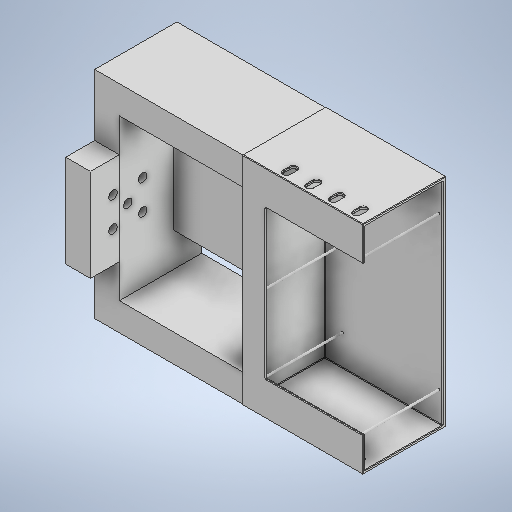
# Autodesk Inventor part: Intake_I2D_Bottom
Saved by Autodesk Inventor 2025 (Build 290162010, 162A)
## iProperties
Created: 2024-10-13
Part Number: Intake_I2D_Bottom
Material: Generic
Document SubType Name: Modeling
Designer: dcfam
Density: 1 g/cm^3
Appearance: Default
Author: dcfam
Autodesk Inventor part; units mm, degrees
ref_plane "YZ Plane" through (0, 0, 0) normal (1, 0, 0) x (0, 1, 0)
ref_plane "XZ Plane" through (0, 0, 0) normal (0, 1, 0) x (-1, 0, 0)
ref_plane "XY Plane" through (0, 0, 0) normal (0, 0, 1) x (1, 0, 0)
sketch "Sketch1" plane through (0, 0, 0) normal (0, 0, 1) x (1, 0, 0)
  line L0 (-32.5, -58.5) -> (32.5, -58.5)
  line L1 (32.5, -58.5) -> (32.5, 58.5)
  line L2 (32.5, 58.5) -> (-32.5, 58.5)
  line L3 (-32.5, 58.5) -> (-32.5, -58.5)
  line L4 (-32.5, -58.5) -> (32.5, 58.5) construction
  line L5 (32.5, -58.5) -> (-32.5, 58.5) construction
  point P0 (0, 0)
  dimension "d0" = 65
  dimension "d1" = 117
  constraints: 12 end point, 2 midpoint, 2 parallel, 1 horizontal, 1 perpendicular
  measures "d0" distance of L2.end L1.end
  measures "d1" distance of L1.end L0.end
extrude "Extrusion1" add sketch "Sketch1" along normal blind 2
sketch "Sketch2" plane through (0, 0, 2) normal (0, 0, 1) x (1, 0, 0)
  line L0 (32.5, -58.5) -> (32.5, 58.5) projected
  line L1 (32.5, 58.5) -> (-32.5, 58.5) projected
  line L2 (-32.5, 58.5) -> (-32.5, -58.5) projected
  line L3 (-32.5, -58.5) -> (32.5, -58.5) projected
  line L4 (31, 57) -> (-31, 57)
  line L5 (-31, 57) -> (-31, -57)
  line L6 (-31, -57) -> (26, -57)
  line L7 (26, -57) -> (32.5, -57)
  line L8 (32.5, -58.5) -> (32.5, 58.5) projected
  line L9 (32.5, -57) -> (32.5, -58.5)
  line L10 (31, 57) -> (32.5, 57)
  line L11 (32.5, 57) -> (32.5, 58.5)
  line L12 (32.5, 58.5) -> (-32.5, 58.5)
  line L13 (-32.5, 58.5) -> (-32.5, -58.5)
  line L14 (-32.5, -58.5) -> (32.5, -58.5)
  point P0 (0, 0)
  dimension "d4" = 1.5
  constraints: 20 end point, 4 perpendicular, 2 collinear, 2 point on line, 1 horizontal, 2 other
  measures "d4" distance between parallel lines of L3 L6
extrude "Extrusion2" add sketch "Sketch2" along normal blind 43 contours L3 L2 L1 L0 L10 L4 L5 L6 L7
sketch "Sketch3" plane through (0, 0, 45) normal (0, 0, 1) x (1, 0, 0)
  line L0 (-32.5, -58.5) -> (32.5, -58.5) projected
  line L1 (32.5, 58.5) -> (-32.5, 58.5) projected
  line L2 (-32.5, -58.5) -> (32.5, -58.5)
  line L3 (32.5, -58.5) -> (32.5, 58.5)
  line L4 (32.5, 58.5) -> (-32.5, 58.5)
  line L5 (-32.5, 58.5) -> (-32.5, -58.5)
  point P0 (0, 0)
  constraints: 8 end point, 2 parallel, 1 horizontal, 1 perpendicular
extrude "Extrusion3" add sketch "Sketch3" against normal blind 1
sketch "Sketch4" plane through (0, 0, 45) normal (0, 0, 1) x (1, 0, 0)
  line L0 (20, -40) -> (-20, -40)
  line L1 (-20, -40) -> (-20, 40)
  line L2 (-20, 40) -> (20, 40)
  line L3 (20, -40) -> (-20, 40) construction
  line L4 (-20, -40) -> (20, 40) construction
  line L5 (20, -40) -> (32.5, -40)
  line L6 (32.5, 57) -> (32.5, -57) projected
  line L7 (20, 40) -> (32.5, 40)
  line L8 (32.5, 40) -> (32.5, -40)
  line L9 (32.5, -40) -> (32.5, 40)
  point P0 (0, 0)
  point P1 (32.5, 40)
  dimension "d9" = 40
  dimension "d10" = 80
  constraints: 18 end point, 3 horizontal, 2 midpoint, 2 perpendicular, 1 collinear, 1 parallel, 1 point on line
  measures "d9" distance of L1.end L2.end
  measures "d10" distance of L0.end L1.end
extrude "Extrusion4" cut sketch "Sketch4" against normal blind 10.525
sketch "Sketch5" plane through (-32.5, 58.5, 0) normal (0, 1, 0) x (1, 0, 0)
  arc A0 (59.7, -37.9468) -> (56.3, -37.9468) centre (58, -37.7472) ccw
  line L0 (56.3, -37.9468) -> (56.3, -41.0568)
  line L1 (56.3, -41.0568) -> (56.3, -37.9468)
  line L2 (56.3, -39.5018) -> (63.0274, -39.5018) construction
  arc A1 (56.3, -41.0568) -> (59.7, -41.0568) centre (58, -41.2563) ccw
  line L3 (58, -41.2563) -> (58, -37.7472) construction
  line L4 (59.7, -37.9468) -> (59.7, -41.0568)
  line L5 (65, 0) -> (65, -45) construction
  line L6 (65, 0) -> (0, 0) construction
  line L7 (0, 0) -> (0, -45) construction
  line L8 (65, -45) -> (0, -45) construction
  arc A2 (43.7, -41.0568) -> (47.1, -41.0568) centre (45.4, -41.2563) ccw
  line L9 (47.1, -37.9468) -> (47.1, -41.0568)
  arc A3 (47.1, -37.9468) -> (43.7, -37.9468) centre (45.4, -37.7472) ccw
  line L10 (43.7, -37.9468) -> (43.7, -41.0568)
  arc A4 (31.1, -41.0568) -> (34.5, -41.0568) centre (32.8, -41.2563) ccw
  line L11 (34.5, -37.9468) -> (34.5, -41.0568)
  arc A5 (34.5, -37.9468) -> (31.1, -37.9468) centre (32.8, -37.7472) ccw
  line L12 (31.1, -37.9468) -> (31.1, -41.0568)
  arc A6 (18.5, -41.0568) -> (21.9, -41.0568) centre (20.2, -41.2563) ccw
  line L13 (21.9, -37.9468) -> (21.9, -41.0568)
  arc A7 (21.9, -37.9468) -> (18.5, -37.9468) centre (20.2, -37.7472) ccw
  line L14 (18.5, -37.9468) -> (18.5, -41.0568)
  line L15 (58, -42.968) -> (20.2, -42.968) construction
  line L16 (39.1, -42.968) -> (39.1, -55.668) construction
  point P0 (32.5, 0)
  point P1 (21.9, -37.9468)
  point P2 (18.5, -41.0568)
  point P3 (21.9, -41.0568)
  point P4 (34.5, -37.9468)
  point P5 (31.1, -41.0568)
  point P6 (34.5, -41.0568)
  point P7 (47.1, -37.9468)
  point P8 (43.7, -41.0568)
  point P9 (47.1, -41.0568)
  point P10 (59.7, -37.9468)
  point P11 (56.3, -41.0568)
  point P12 (59.7, -41.0568)
  dimension "d13" = 3.4
  dimension "d14" = 1.7117
  dimension "d15" = 3.11
  dimension "d16" = 3.11
  dimension "d19" = 12.6
  dimension "d24" = 2.032
  dimension "d37" = 12.7
  dimension "d47" = 32.6288
  dimension "d48" = 1.9726
  dimension "d49" = 1.9726
  dimension "d50" = 35.7388
  dimension "d51" = 1.9726
  dimension "d52" = 35.7388
  dimension "d53" = 5.3726
  dimension "d54" = 32.6288
  dimension "d55" = 14.5726
  dimension "d56" = 35.7388
  dimension "d57" = 14.5726
  dimension "d58" = 35.7388
  dimension "d59" = 17.9726
  dimension "d60" = 32.6288
  dimension "d61" = 27.1726
  dimension "d62" = 35.7388
  dimension "d63" = 27.1726
  dimension "d64" = 35.7388
  dimension "d65" = 30.5726
  dimension "d66" = 32.6288
  dimension "d67" = 39.7726
  dimension "d68" = 35.7388
  dimension "d69" = 39.7726
  dimension "d70" = 35.7388
  dimension "d71" = 43.1726
  dimension "d84" = 5.3
  constraints: 26 end point, 18 point on circle, 8 centre point, 5 symmetric about line, 4 point on line, 3 vertical, 2 horizontal, 2 midpoint, 1 coincident, 1 tangent, 43 other
  measures "d13" distance of A0.start L0.start
  measures "d14" radius of A0
  measures "d15" distance of L0.start L0.end
  measures "d16" distance of L0.end L1.end
  measures "d19" distance of L3.start A2.centre
  measures "d24" distance from line of L8 L15.start
  measures "d37" distance of L16.start L16.end
  measures "d49" distance from line of L2.end L5
  measures "d84" distance between parallel lines of L5 L4
extrude "Extrusion5" cut sketch "Sketch5" against normal blind 25.4
sketch "Sketch6" plane through (-32.5, -58.5, 0) normal (0, -1, 0) x (1, 0, 0)
  circle A0 centre (57.992, 40.3585) radius 1.9625
  line L0 (0, 0) -> (0, 45) projected
  line L1 (0, 0) -> (65, 0) projected
  line L2 (65, 0) -> (65, 45) projected
  line L3 (0, 45) -> (65, 45) projected
  circle A1 centre (49.991, 40.3585) radius 1.9625
  circle A2 centre (41.99, 40.3585) radius 1.9625
  circle A3 centre (33.989, 40.3585) radius 1.9625
  line L4 (33.989, 42.321) -> (57.992, 42.321) construction
  line L5 (45.9905, 42.321) -> (45.9905, 58.396) construction
  point P0 (32.5, 0)
  dimension "d27" = 3.925
  dimension "d30" = 8.001
  dimension "d35" = 2.679
  dimension "d36" = 16.075
  dimension "d87" = 7.008
  constraints: 4 end point, 2 centre point, 2 horizontal, 2 vertical alignment, 1 coincident, 1 midpoint, 1 vertical, 10 other
  measures "d30" distance of point (57.992, 40.358) A1.centre
  measures "d35" distance between parallel lines of L3 L4
  measures "d36" distance of L5.start L5.end
  measures "d87" distance from line of L2 point (57.992, 40.358)
extrude "Extrusion6" cut sketch "Sketch6" against normal blind 25.4 contours A0 | A1 | A2 | A3
chamfer "Chamfer1" distance 0.5 angle 45 8 edges at (23.5295, -57, 40.3585) (15.5285, -57, 40.3585) (7.5275, -57, 40.3585) (-0.4735, -57, 40.3585) (-0.4735, -58.5, 40.3585) (7.5275, -58.5, 40.3585) (15.5285, -58.5, 40.3585) (23.5295, -58.5, 40.3585)
fillet "Fillet1" radius 0.3 100 edges at (0, -58.5, 45) (15.5285, -57.5, 40.3585) (15.0285, -57, 40.3585) (23.5295, -58, 40.3585) (23.5295, -57.5, 40.3585) (23.0295, -58.5, 40.3585) (7.0275, -58.5, 40.3585) (23.0295, -57, 40.3585) (7.0275, -57, 40.3585) (-0.4735, -58, 40.3585) (-0.4735, -57.5, 40.3585) (-0.9735, -58.5, 40.3585) (-0.9735, -57, 40.3585) (32.5, -57, 23) (32.5, -58.5, 22.5) (0.75, -57, 44) (0.75, -57, 2) (0, -58.5, 0) (-31, -57, 23) (-32.5, -58.5, 22.5) (7.5275, -58, 40.3585) (15.5285, -58, 40.3585) (15.0285, -58.5, 40.3585) (7.5275, -57.5, 40.3585) (-20, 0, 44) (-20, 0, 45) (-31, 0, 44) (-32.5, 0, 45) (-32.5, 0, 0) (0.75, 57, 44) (0.75, 57, 2) (-31, 57, 23) (0, 58.5, 45) (0, 58.5, 0) (-32.5, 58.5, 22.5) (32.5, 57, 23) (32.5, 49.25, 45) (32.5, 58.5, 22.5) (32.5, 48.5, 44) (32.5, -48.5, 44) (32.5, 0, 0) (32.5, 0, 2) (32.5, -49.25, 45) (6.25, -40, 45) (6.25, -40, 44) (32.5, -40, 44.5) (-20, -40, 44.5) (-31, 0, 2) (32.5, 40, 44.5) (-20, 40, 44.5) (6.25, 40, 45) (6.25, 40, 44) (27.2, 58.5, 39.5018) (23.8, 57, 39.5018) (27.2, 57, 39.5018) (25.5, 57, 36.0355) (25.5, 57, 42.968) (23.8, 58.5, 39.5018) (23.8, 57.75, 37.9468) (25.5, 58.5, 36.0355) (27.2, 57.75, 37.9468) (27.2, 57.75, 41.0568) (25.5, 58.5, 42.968) (23.8, 57.75, 41.0568) (-10.6, 58.5, 39.5018) (-10.6, 57, 39.5018) (-14, 57, 39.5018) (-12.3, 57, 36.0355) (-10.6, 57.75, 41.0568) (-10.6, 57.75, 37.9468) (-12.3, 58.5, 36.0355) (-14, 58.5, 39.5018) (-14, 57.75, 37.9468) (-14, 57.75, 41.0568) (-12.3, 58.5, 42.968) (-12.3, 57, 42.968) (14.6, 57, 39.5018) (12.9, 57, 42.968) (11.2, 57, 39.5018) (12.9, 57, 36.0355) (12.9, 58.5, 36.0355) (12.9, 58.5, 42.968) (11.2, 57.75, 41.0568) (11.2, 58.5, 39.5018) (11.2, 57.75, 37.9468) (14.6, 58.5, 39.5018) (14.6, 57.75, 37.9468) (14.6, 57.75, 41.0568) (-1.4, 57, 39.5018) (0.3, 57, 36.0355) (2, 57, 39.5018) (2, 57.75, 41.0568) (2, 57.75, 37.9468) (0.3, 58.5, 36.0355) (-1.4, 57.75, 41.0568) (-1.4, 57.75, 37.9468) (-1.4, 58.5, 39.5018) (0.3, 58.5, 42.968) (2, 58.5, 39.5018) (0.3, 57, 42.968)
sketch "Sketch11" plane through (-32.5, -58.2, 0.3) normal (-1, 0, 0) x (0, 0, 1)
  line L0 (44, 97.9) -> (44, 18.5) construction
  line L1 (44, 58.2) -> (-0.3, 58.2) construction
  line L2 (0, 0) -> (44.4, 0) construction
  line L3 (22.2, 0) -> (22.2, 116.4) construction
  line L4 (0, 116.4) -> (44.4, 116.4) construction
  line L5 (15, 83.2) -> (0, 83.2)
  line L6 (0, 83.2) -> (0, 33.2)
  line L7 (0, 33.2) -> (15, 33.2)
  line L8 (15, 33.2) -> (15, 83.2)
  line L9 (15, 83.2) -> (0, 33.2) construction
  line L10 (0, 83.2) -> (15, 33.2) construction
  line L11 (0, 0) -> (0, 116.4) projected
  line L12 (0, 15) -> (44.4, 15)
  line L13 (44.4, 15) -> (44.4, 0)
  line L14 (44.4, 0) -> (0, 0)
  line L15 (0, 0) -> (0, 15)
  line L16 (0, 15) -> (44.4, 0) construction
  line L17 (44.4, 15) -> (0, 0) construction
  line L18 (0, 116.4) -> (44.4, 116.4) construction
  line L19 (0, 101.4) -> (44.4, 101.4)
  line L20 (44.4, 101.4) -> (44.4, 116.4)
  line L21 (44.4, 116.4) -> (0, 116.4)
  line L22 (0, 116.4) -> (0, 101.4)
  point P0 (7.5, 58.2)
  point P1 (22.2, 7.5)
  dimension "d111" = 50
  dimension "d113" = 15
  dimension "d115" = 15
  constraints: 38 end point, 7 midpoint, 4 parallel, 4 symmetric about line, 3 collinear, 3 horizontal, 2 perpendicular, 2 point on line
  measures "d111" distance of L6.end L5.end
  measures "d113" distance of L6.end L7.end
  measures "d115" distance of L12.end L13.end
extrude "Extrusion10" add sketch "Sketch11" along normal blind 80
sketch "Sketch12" plane through (-32.5, -25, 15.3) normal (0, 0, 1) x (1, 0, 0)
  line L0 (0, 50) -> (0, 0) projected
  line L1 (0, 50) -> (-80, 50) projected
  line L2 (-80, 0) -> (-80, 50) projected
  line L3 (0, 0) -> (-80, 0) projected
  line L4 (0, 83.2) -> (0, 68.2) projected
  line L5 (0, 83.2) -> (-80, 83.2) projected
  line L6 (-80, 68.2) -> (-80, 83.2) projected
  line L7 (0, 68.2) -> (-80, 68.2) projected
  line L8 (0, -18.2) -> (0, -33.2) projected
  line L9 (0, -18.2) -> (-80, -18.2) projected
  line L10 (-80, -33.2) -> (-80, -18.2) projected
  line L11 (0, -33.2) -> (-80, -33.2) projected
  arc A0 (12.2, -14.7) -> (12.8, -15.3) centre (12.8, -14.7) ccw projected
  line L12 (12.2, 64.7) -> (12.2, -14.7) projected
  arc A1 (12.8, 65.3) -> (12.2, 64.7) centre (12.8, 64.7) ccw projected
  line L13 (64.7, 65.3) -> (12.8, 65.3) projected
  line L14 (64.7, 83.2) -> (64.7, 65.3) projected
  line L15 (0.3, 83.2) -> (64.7, 83.2) projected
  line L16 (0.3, -33.2) -> (0.3, 83.2) projected
  line L17 (64.7, -33.2) -> (0.3, -33.2) projected
  line L18 (64.7, -15.3) -> (64.7, -33.2) projected
  line L19 (12.8, -15.3) -> (64.7, -15.3) projected
  line L20 (64.7, 81.7) -> (64.7, -31.7) projected
  line L21 (1.8, 81.7) -> (64.7, 81.7) projected
  line L22 (1.8, -31.7) -> (1.8, 81.7) projected
  line L23 (64.7, -31.7) -> (1.8, -31.7) projected
  line L24 (-60, 0) -> (-60, 50) construction
  line L25 (-80, 0) -> (-73.334, 0)
  line L26 (-73.334, 0) -> (-73.334, 50)
  line L27 (-73.334, 50) -> (-80, 50)
  line L28 (-80, 50) -> (-80, 0)
  point P0 (32.5, 25)
  point P1 (-73.334, 0)
  dimension "d118" = 20
  dimension "d119" = 6.666
  constraints: 10 end point, 3 point on line, 2 parallel, 2 perpendicular, 1 horizontal
  measures "d118" distance between parallel lines of L2 L24
  measures "d119" distance of L27.end L26.end
extrude "Extrusion11" add sketch "Sketch12" along normal blind 45 contours L26 L3 L2 L1
sketch "Sketch15" plane through (-32.5, -43.2, 44.7) normal (0, 1, 0) x (1, 0, 0)
  line L0 (0, 0) -> (-80, 0) construction
  line L1 (-73.334, 0) -> (-73.334, 44.4) construction
  line L2 (0, 44.4) -> (-80, 44.4) construction
  line L3 (-80, 0) -> (-80, 44.4) construction
  line L4 (-66.668, 0) -> (-66.668, 39.243) construction
  line L5 (-73.334, 0) -> (-66.668, 0)
  line L6 (-66.668, 0) -> (-66.668, 39.243)
  line L7 (-66.668, 39.243) -> (-73.334, 39.243)
  line L8 (-73.334, 39.243) -> (-73.334, 0)
  point P0 (32.5, 44.7)
  point P1 (0, 39.243)
  dimension "d130" = 6.666
  dimension "d131" = 6.666
  constraints: 12 end point, 2 parallel, 2 point on line, 2 vertical, 1 horizontal, 1 perpendicular, 2 other
  measures "d130" distance between parallel lines of L3 L1
  measures "d131" distance between parallel lines of L4 L1
extrude "Extrusion14" add sketch "Sketch15" along normal blind 68.2
sketch "Sketch18" plane through (-32.5, 43.2, 0.3) normal (0, -1, 0) x (1, 0, 0)
  line L0 (0, 0) -> (-80, 0) construction
  line L1 (-73.334, 0) -> (-73.334, 44.4) construction
  line L2 (0, 44.4) -> (-80, 44.4) construction
  line L3 (-80, 0) -> (-80, 44.4) construction
  line L4 (-66.668, 0) -> (-66.668, 44.4) construction
  line L5 (-73.334, 0) -> (-66.668, 0)
  line L6 (-66.668, 0) -> (-66.668, 44.4)
  line L7 (-66.668, 44.4) -> (-73.334, 44.4)
  line L8 (-73.334, 44.4) -> (-73.334, 0)
  point P0 (32.5, -0.3)
  point P1 (0, 39.243)
  dimension "d138" = 6.666
  dimension "d140" = 6.666
  constraints: 12 end point, 2 parallel, 2 point on line, 2 vertical, 1 horizontal, 1 perpendicular, 3 other
  measures "d138" distance between parallel lines of L3 L1
  measures "d140" distance between parallel lines of L4 L1
extrude "Extrusion17" add sketch "Sketch18" along normal blind 60
sketch "Sketch19" plane through (-112.5, -58.2, 0.3) normal (-1, 0, 0) x (0, 0, 1)
  line L0 (15, 83.2) -> (15, 33.2) construction
  line L1 (2.54, 35.74) -> (2.54, 80.66) construction
  line L2 (57.46, 35.74) -> (2.54, 35.74) construction
  line L3 (57.46, 80.66) -> (57.46, 35.74) construction
  line L4 (2.54, 80.66) -> (57.46, 80.66) construction
  line L5 (50.1093, 35.74) -> (50.1093, 80.66) construction
  circle A0 centre (47.8593, 50.2) radius 2.25
  line L6 (2.54, 58.2) -> (57.46, 58.2) construction
  circle A1 centre (47.8593, 66.2) radius 2.25
  line L7 (39.8593, 35.74) -> (39.8593, 80.66) construction
  circle A2 centre (31.8593, 50.2) radius 2.25
  circle A3 centre (31.8593, 66.2) radius 2.25
  circle A4 centre (39.8593, 58.2) radius 2.25
  point P0 (-0.3, 58.2)
  dimension "d152" = 4.5
  dimension "d153" = 16
  dimension "d154" = 16
  dimension "d155" = 4.5
  constraints: 6 end point, 5 centre point, 4 point on line, 3 midpoint, 3 symmetric about line, 2 perpendicular, 1 tangent, 3 other
  measures "d152" diameter of A0
  measures "d153" distance of A1.centre A0.centre
  measures "d154" distance of A0.centre A2.centre
  measures "d155" diameter of A4
extrude "Extrusion18" cut sketch "Sketch19" against normal blind 60
chamfer "Chamfer4" distance 0.762 angle 45 5 edges at (-112.5, 8, 29.9093) (-112.5, 0, 37.9093) (-112.5, -8, 29.9093) (-112.5, -8, 45.9093) (-112.5, 8, 45.9093)
sketch "Sketch20" plane through (0, 0, 44) normal (0, 0, -1) x (-1, 0, 0)
  line L0 (0, 0) -> (-41.559, 0) construction
  circle A0 centre (-30.5926, -41.1687) radius 0.5
  circle A1 centre (-30.5926, 41.1687) radius 0.5
  circle A2 centre (22.3359, 40.6687) radius 0.5
  circle A3 centre (22.1062, 0) radius 0.5
  circle A4 centre (21.6062, -40.6687) radius 0.5
  dimension "d161" = 1
  constraints: 5 centre point, 2 end point, 1 horizontal, 1 symmetric about line, 1 other
  measures "d161" diameter of A0
extrude "Extrusion19" add sketch "Sketch20" along normal blind 43.942
thicken "Thicken1" operation add thickness 6.6548 both sides no extend neighbours no toward (1, 0, 0) faces at (-105.834, 2.4872, 56.9813)
thicken "Thicken2" operation add thickness 6.6548 both sides no extend neighbours no toward (-1, 0, 0) faces at (-105.834, -31.0667, 31.619)
thicken "Thicken3" operation add thickness 6.6548 both sides no extend neighbours no toward (-1, 0, 0) faces at (-105.834, 31.0667, 15.1)
thicken "Thicken4" operation add thickness 5.157 both sides no extend neighbours no toward (0, 0, -1) faces at (-103.6083, -37.1333, 5.457)
body "Solid1"
